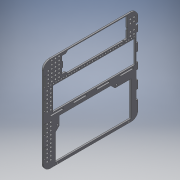
# Autodesk Inventor part: TrayPanelE
Saved by Autodesk Inventor 2017 (Build 210142000, 142)
## iProperties
Created: 2019-06-22
Part Number: TrayPanelE
Material: Generic
Document SubType Name: Modeling
Designer: DDeGo
Density: 1 g/cm^3
Appearance: Default
Author: DDeGo
Autodesk Inventor part; units mm, degrees
ref_plane "YZ Plane" through (0, 0, 0) normal (1, 0, 0) x (0, 1, 0)
ref_plane "XZ Plane" through (0, 0, 0) normal (0, 1, 0) x (-1, 0, 0)
ref_plane "XY Plane" through (0, 0, 0) normal (0, 0, 1) x (1, 0, 0)
sketch "Block1" plane through (0, 0, 0) normal (0, 0, 1) x (1, 0, 0)
  circle A0 centre (145, 9.5) radius 1.5
  circle A1 centre (31, 19.5) radius 1.5
  circle A2 centre (31, 83.5) radius 1.5
  circle A3 centre (169, 83.5) radius 1.5
  line L0 (27, 29.5) -> (27, 80.5)
  line L1 (27, 80.5) -> (173, 80.5)
  line L2 (173, 80.5) -> (173, 13.5)
  line L3 (173, 13.5) -> (142, 13.5)
  line L4 (142, 13.5) -> (134, 5.5)
  line L5 (134, 5.5) -> (34, 5.5)
  line L6 (34, 5.5) -> (34, 22.5)
  line L7 (34, 22.5) -> (27, 29.5)
  point P0 (93.25, 35.7812)
sketch "Sketch1" plane through (0, 0, 0) normal (1, 0, 0) x (0, 1, 0)
  line L0 (46.5, 144.8143) -> (46.5, 184.0143) construction
  line L1 (46.5, 184.0143) -> (162.5, 184.0143)
  line L2 (162.5, 184.0143) -> (162.5, 144.8143)
  line L3 (170, 185.4143) -> (13, 185.4143)
  arc A0 (13, 185.4143) -> (0, 172.4143) centre (13, 172.4143) ccw
  line L4 (0, 172.4143) -> (0, 15.4143)
  arc A1 (0, 15.4143) -> (13, 2.4143) centre (13, 15.4143) ccw
  line L5 (13, 2.4143) -> (170, 2.4143)
  arc A2 (170, 2.4143) -> (183, 15.4143) centre (170, 15.4143) ccw
  line L6 (183, 15.4143) -> (183, 172.4143)
  arc A3 (183, 172.4143) -> (170, 185.4143) centre (170, 172.4143) ccw
  line L7 (186.5, 14.4143) -> (186.5, 173.4143) projected
  arc A4 (186.5, 173.4143) -> (171, 188.9143) centre (171, 173.4143) ccw projected
  line L8 (171, 188.9143) -> (12, 188.9143) projected
  arc A5 (12, 188.9143) -> (-3.5, 173.4143) centre (12, 173.4143) ccw projected
  line L9 (-3.5, 173.4143) -> (-3.5, 14.4143) projected
  arc A6 (-3.5, 14.4143) -> (12, -1.0857) centre (12, 14.4143) ccw projected
  line L10 (12, -1.0857) -> (171, -1.0857) projected
  arc A7 (171, -1.0857) -> (186.5, 14.4143) centre (171, 14.4143) ccw projected
  arc A8 (46.5, 184.0143) -> (46.1505, 183.8718) centre (46.5, 183.5143) ccw
  line L11 (46.1505, 183.8718) -> (42.3495, 180.1567)
  arc A9 (42, 180.0143) -> (42.3495, 180.1567) centre (42, 180.5143) ccw
  line L12 (42, 180.0143) -> (35.5, 180.0143)
  arc A10 (35.5, 180.0143) -> (34.5, 179.0143) centre (35.5, 179.0143) ccw
  line L13 (34.5, 179.0143) -> (34.5, 170.4143)
  arc A11 (34.5, 170.4143) -> (35.5, 169.4143) centre (35.5, 170.4143) ccw
  line L14 (35.5, 169.4143) -> (37, 169.4143)
  line L15 (37, 159.4143) -> (35.5, 159.4143)
  arc A12 (35.5, 159.4143) -> (34.5, 158.4143) centre (35.5, 158.4143) ccw
  line L16 (34.5, 158.4143) -> (34.5, 149.8143)
  arc A13 (34.5, 149.8143) -> (35.5, 148.8143) centre (35.5, 149.8143) ccw
  line L17 (35.5, 148.8143) -> (42, 148.8143)
  arc A14 (42.3495, 148.6718) -> (42, 148.8143) centre (42, 148.3143) ccw
  line L18 (42.3495, 148.6718) -> (46.1505, 144.9567)
  arc A15 (46.1505, 144.9567) -> (46.5, 144.8143) centre (46.5, 145.3143) ccw
  line L19 (37, 169.4143) -> (37, 159.4143)
  line L20 (177.5, 93.9143) -> (18.5, 93.9143)
  line L21 (18.5, 93.9143) -> (18.5, 138.6143)
  line L22 (18.5, 138.6143) -> (177.5, 138.6143)
  line L23 (177.5, 138.6143) -> (177.5, 93.9143)
  line L24 (156.5, 144.8143) -> (156.5, 141.3143)
  line L25 (156.5, 141.3143) -> (155, 141.3143)
  line L26 (155, 141.3143) -> (155, 144.8143)
  line L27 (162.5, 144.8143) -> (156.5, 144.8143)
  line L28 (155, 144.8143) -> (46.5, 144.8143)
  line L29 (37, 164.4143) -> (41, 164.4143) construction
  circle A16 centre (41, 164.4143) radius 1.5 construction
  line L30 (37.5, 154.4143) -> (44.5, 154.4143) construction
  line L31 (44.5, 154.4143) -> (44.5, 174.4143) construction
  line L32 (44.5, 174.4143) -> (37.5, 174.4143) construction
  line L33 (37.5, 174.4143) -> (37.5, 154.4143) construction
  line L34 (37.5, 154.4143) -> (44.5, 174.4143) construction
  line L35 (44.5, 154.4143) -> (37.5, 174.4143) construction
  line L36 (169.5, 77.9143) -> (138.5, 77.9143)
  circle A17 centre (141.5, 81.9143) radius 2.25
  line L37 (138.5, 77.9143) -> (130.5, 85.9143)
  line L38 (130.5, 85.9143) -> (30.5, 85.9143)
  circle A18 centre (27.5, 71.9143) radius 2.25
  line L39 (30.5, 85.9143) -> (30.5, 68.9143)
  line L40 (30.5, 68.9143) -> (23.5, 61.9143)
  line L41 (23.5, 61.9143) -> (23.5, 10.9143)
  circle A19 centre (27.5, 7.9143) radius 2.25
  line L42 (23.5, 10.9143) -> (169.5, 10.9143)
  circle A20 centre (165.5, 7.9143) radius 2.25
  line L43 (169.5, 10.9143) -> (169.5, 77.9143)
  point P0 (46.5, 164.4143)
  point P1 (-6.081, 1.5)
  dimension "d3" = 183
  dimension "d5" = 13
  dimension "d10" = 10.6
  dimension "d11" = 10.6
  dimension "d12" = 10
  dimension "d17" = 4
  dimension "d18" = 0.5
  dimension "d19" = 1
  dimension "d55" = 183
  dimension "d57" = 3.5
  dimension "d63" = 18.5
  dimension "d64" = 91.5
  dimension "d65" = 44.7
  dimension "d66" = 159
  dimension "d67" = 3.5
  dimension "d85" = 20.5
  dimension "d86" = 1.4
  dimension "d87" = 116
  dimension "d88" = 4
  dimension "d89" = 3.5
  dimension "d90" = 6
  dimension "d91" = 1.5
  dimension "d92" = 12
  dimension "d93" = 2.5
  dimension "d94" = 4.5
  dimension "d95" = 4.5
  dimension "d96" = 3
  dimension "d97" = 7
  dimension "d98" = 4
  dimension "d99" = 20
  dimension "d103" = 122
  constraints: 80 end point, 25 tangent, 24 point on circle, 17 centre point, 11 horizontal, 9 equal radius, 8 perpendicular, 6 vertical, 4 midpoint, 4 parallel, 1 coincident, 1 collinear, 18 other
  measures "d3" distance between parallel lines of L3 L5
  measures "d5" radius of A0
  measures "d10" distance between parallel lines of L12 L14
  measures "d11" distance between parallel lines of L17 L15
  measures "d12" distance between parallel lines of L14 L15
  measures "d17" distance between parallel lines of L1 L12
  measures "d18" radius of A14
  measures "d19" radius of A13
  measures "d55" distance between parallel lines of L6 L4
  measures "d57" distance between parallel lines of L9 L4
  measures "d63" distance between parallel lines of L4 L21
  measures "d64" distance between parallel lines of L5 L20
  measures "d65" distance between parallel lines of L22 L20
  measures "d66" distance between parallel lines of L23 L21
  measures "d67" distance between parallel lines of L10 L5
  measures "d85" distance between parallel lines of L6 L2
  measures "d86" distance between parallel lines of L3 L1
  measures "d87" distance between parallel lines of L2 L0
  measures "d88" distance between parallel lines of L17 L28
  measures "d89" distance between parallel lines of L28 L25
  measures "d90" distance between parallel lines of L24 L2
  measures "d91" distance between parallel lines of L26 L24
  measures "d92" distance between parallel lines of L0 L13
  measures "d93" distance between parallel lines of L13 L19
  measures "d94" distance from line of L0 L12.start
  measures "d95" distance from line of L0 L17.end
  measures "d96" diameter of A16
  measures "d97" distance of L30.start L30.end
  measures "d98" distance of L29.start L29.end
  measures "d99" distance of L30.end L31.end
  measures "d103" distance between parallel lines of L13 L24
extrude "Extrusion1" add sketch "Sketch1" along normal blind 2.75 contours A3 L6 A2 L5 A1 L4 A0 L3
sketch "Sketch2" plane through (2.75, 0, 0) normal (1, 0, 0) x (0, 0, -1)
  line L0 (-91.375, 13.5) -> (-88.625, 13.5)
  line L1 (-88.625, 13.5) -> (-88.625, 38.5)
  line L2 (-88.625, 38.5) -> (-91.375, 38.5)
  line L3 (-91.375, 38.5) -> (-91.375, 13.5)
  line L4 (-91.375, 58.5) -> (-88.625, 58.5)
  line L5 (-88.625, 58.5) -> (-88.625, 83.5)
  line L6 (-88.625, 83.5) -> (-91.375, 83.5)
  line L7 (-91.375, 83.5) -> (-91.375, 58.5)
  line L8 (-91.375, 103.5) -> (-88.625, 103.5)
  line L9 (-88.625, 103.5) -> (-88.625, 128.5)
  line L10 (-88.625, 128.5) -> (-91.375, 128.5)
  line L11 (-91.375, 128.5) -> (-91.375, 103.5)
  line L12 (-91.375, 148.5) -> (-88.625, 148.5)
  line L13 (-88.625, 148.5) -> (-88.625, 173.5)
  line L14 (-88.625, 173.5) -> (-91.375, 173.5)
  line L15 (-91.375, 173.5) -> (-91.375, 148.5)
  line L16 (-162, 1.625) -> (-142, 1.625)
  line L17 (-142, 1.625) -> (-142, 4.375)
  line L18 (-142, 4.375) -> (-162, 4.375)
  line L19 (-162, 4.375) -> (-162, 1.625)
  line L20 (-122, 1.625) -> (-102, 1.625)
  line L21 (-102, 1.625) -> (-102, 4.375)
  line L22 (-102, 4.375) -> (-122, 4.375)
  line L23 (-122, 4.375) -> (-122, 1.625)
  line L24 (-82, 1.625) -> (-62, 1.625)
  line L25 (-62, 1.625) -> (-62, 4.375)
  line L26 (-62, 4.375) -> (-82, 4.375)
  line L27 (-82, 4.375) -> (-82, 1.625)
  line L28 (-42, 1.625) -> (-22, 1.625)
  line L29 (-22, 1.625) -> (-22, 4.375)
  line L30 (-22, 4.375) -> (-42, 4.375)
  line L31 (-42, 4.375) -> (-42, 1.625)
  line L32 (-15.4143, 183) -> (-172.4143, 183) projected
  line L33 (-172.4143, 0) -> (-15.4143, 0) projected
  line L34 (-185.4143, 170) -> (-185.4143, 13) projected
  point P0 (0, 0)
  point P1 (-90, 128.5)
  point P2 (-142, 3)
  dimension "d22" = 25
  dimension "d23" = 2.75
  dimension "d24" = 9.5
  dimension "d29" = 90
  dimension "d30" = 2.75
  dimension "d31" = 3
  dimension "d32" = 22
  dimension "d36" = 20
  dimension "d37" = 23.4143
  dimension "d38" = 9.125
  dimension "d41" = 45
  dimension "d42" = 45
  dimension "d43" = 45
  dimension "d44" = 40
  dimension "d45" = 40
  dimension "d46" = 40
  constraints: 64 end point, 16 parallel, 12 point on line, 8 horizontal, 8 perpendicular, 6 collinear, 2 midpoint
  measures "d22" distance of L2.end L0.start
  measures "d23" distance of L13.end L14.end
  measures "d24" distance between parallel lines of L14 L32
  measures "d29" horizontal distance of point (0, 0) point (-90, 128.5)
  measures "d30" distance of L18.end L16.start
  measures "d31" vertical distance of point (0, 0) point (-142, 3)
  measures "d32" horizontal distance of L29.end point (0, 0)
  measures "d36" distance of L17.end L18.end
  measures "d37" distance between parallel lines of L34 L19
  measures "d38" distance between parallel lines of L22 L0
  measures "d41" distance of L10.end L14.end
  measures "d42" distance of L6.end L10.end
  measures "d43" distance of L2.end L6.end
  measures "d44" distance of L25.end L29.end
  measures "d45" distance of L21.end L25.end
  measures "d46" distance of L17.end L21.end
extrude "Extrusion2" cut sketch "Sketch2" against normal blind 10
sketch "Sketch3" plane through (2.75, 0, 0) normal (1, 0, 0) x (0, 0, -1)
  line L0 (-15.4143, 183) -> (-172.4143, 183) projected
  line L1 (-114, 183) -> (-96, 183)
  line L2 (-96, 183) -> (-96, 179.5)
  line L3 (-96, 179.5) -> (-114, 179.5)
  line L4 (-114, 179.5) -> (-114, 183)
  line L5 (-129, 183) -> (-147, 183)
  line L6 (-147, 183) -> (-147, 179.5)
  line L7 (-147, 179.5) -> (-129, 179.5)
  line L8 (-129, 179.5) -> (-129, 183)
  line L9 (-84, 183) -> (-66, 183)
  line L10 (-66, 183) -> (-66, 179.5)
  line L11 (-66, 179.5) -> (-84, 179.5)
  line L12 (-84, 179.5) -> (-84, 183)
  line L13 (-51, 183) -> (-33, 183)
  line L14 (-33, 183) -> (-33, 179.5)
  line L15 (-33, 179.5) -> (-51, 179.5)
  line L16 (-51, 179.5) -> (-51, 183)
  line L17 (-91.375, 173.5) -> (-88.625, 173.5) projected
  line L18 (-90, 173.5) -> (-90, 183) construction
  point P0 (0, 0)
  dimension "d47" = 18
  dimension "d48" = 3.5
  dimension "d49" = 6
  dimension "d50" = 15
  dimension "d51" = 6
  dimension "d52" = 15
  constraints: 34 end point, 8 parallel, 8 point on line, 5 perpendicular, 4 horizontal, 3 collinear, 1 midpoint
  measures "d47" distance of L14.end L15.end
  measures "d48" distance of L5.end L6.end
  measures "d49" distance between parallel lines of L12 L18
  measures "d50" distance between parallel lines of L10 L16
  measures "d51" distance between parallel lines of L2 L18
  measures "d52" distance between parallel lines of L8 L4
extrude "Extrusion3" cut sketch "Sketch3" against normal blind 10
sketch "Sketch5" plane through (0, 0, 0) normal (-1, 0, 0) x (0, 0, 1)
  line L0 (172.4143, 183) -> (147, 183) projected
  line L1 (163.0643, 183) -> (158.7643, 183)
  line L2 (158.7643, 183) -> (158.7643, 178.5)
  line L3 (158.7643, 178.5) -> (163.0643, 178.5)
  line L4 (163.0643, 178.5) -> (163.0643, 183)
  line L5 (144.8143, 156.5) -> (144.8143, 162.5) projected
  line L6 (144.8143, 162.5) -> (184.0143, 162.5) projected
  line L7 (163.0643, 162.5) -> (158.7643, 162.5)
  line L8 (158.7643, 162.5) -> (158.7643, 163.5)
  line L9 (158.7643, 163.5) -> (163.0643, 163.5)
  line L10 (163.0643, 163.5) -> (163.0643, 162.5)
  point P0 (0, 0)
  point P1 (160.9143, 178.5)
  point P2 (144.5143, 47.5)
  point P3 (185.4143, 158)
  dimension "d70" = 16.1
  dimension "d71" = 4.3
  dimension "d72" = 4.5
  dimension "d75" = 1
  constraints: 16 end point, 4 parallel, 2 collinear, 2 horizontal, 2 perpendicular, 1 midpoint, 1 point on line, 3 other
  measures "d71" distance between parallel lines of L4 L2
  measures "d72" distance between parallel lines of L0 L3
extrude "Extrusion5" cut sketch "Sketch5" against normal blind 10
sketch "Sketch6" plane through (0, 0, 0) normal (-1, 0, 0) x (0, 0, 1)
  line L0 (178.4143, 176) -> (9.4143, 176) construction
  line L1 (9.4143, 176) -> (9.4143, 7) construction
  line L2 (9.4143, 7) -> (178.4143, 7) construction
  line L3 (178.4143, 7) -> (178.4143, 176) construction
  line L4 (2.4143, 170) -> (2.4143, 13) construction
  line L5 (33, 183) -> (15.4143, 183) construction
  line L6 (185.4143, 13) -> (185.4143, 170) construction
  line L7 (15.4143, 0) -> (172.4143, 0) construction
  circle A0 centre (178.4143, 176) radius 2.05
  circle A1 centre (178.4143, 7) radius 2.05
  circle A2 centre (9.4143, 7) radius 2.05
  circle A3 centre (9.4143, 176) radius 2.05
  point P0 (0, 0)
  dimension "d76" = 7
  dimension "d77" = 7
  dimension "d78" = 7
  dimension "d79" = 7
  dimension "d80" = 4.1
  constraints: 8 end point, 4 centre point, 4 coincident, 3 equal radius, 2 parallel, 1 horizontal, 1 perpendicular
  measures "d76" distance between parallel lines of L4 L1
  measures "d77" distance between parallel lines of L5 L0
  measures "d78" distance between parallel lines of L6 L3
  measures "d79" distance between parallel lines of L7 L2
  measures "d80" diameter of A0
extrude "Extrusion6" [suppressed]
sketch "Sketch7" plane through (0, 0, 0) normal (-1, 0, 0) x (0, 0, 1)
  circle A0 centre (174.9143, 175.5) radius 2
  circle A1 centre (174.9143, 168.5) radius 2
  circle A2 centre (167.9143, 168.5) radius 2
  circle A3 centre (167.9143, 175.5) radius 2
  circle A4 centre (153.9143, 175.5) radius 2
  circle A5 centre (153.9143, 168.5) radius 2
  circle A6 centre (146.9143, 175.5) radius 2
  circle A7 centre (146.9143, 168.5) radius 2
  circle A8 centre (141.7643, 175.5) radius 1.5
  circle A9 centre (141.7643, 170.4697) radius 1.5
  circle A10 centre (141.7643, 165.4394) radius 1.5
  circle A11 centre (141.7643, 160.4091) radius 1.5
  circle A12 centre (141.7643, 150.3485) radius 1.5
  circle A13 centre (141.7643, 145.3182) radius 1.5
  circle A14 centre (141.7643, 140.2879) radius 1.5
  circle A15 centre (141.7643, 135.2576) radius 1.5
  circle A16 centre (141.7643, 130.2273) radius 1.5
  circle A17 centre (141.7643, 125.197) radius 1.5
  circle A18 centre (141.7643, 120.1667) radius 1.5
  circle A19 centre (141.7643, 115.1364) radius 1.5
  circle A20 centre (141.7643, 110.1061) radius 1.5
  circle A21 centre (141.7643, 105.0758) radius 1.5
  circle A22 centre (141.7643, 100.0455) radius 1.5
  circle A23 centre (141.7643, 95.0152) radius 1.5
  circle A24 centre (141.7643, 89.9848) radius 1.5
  circle A25 centre (141.7643, 84.9545) radius 1.5
  circle A26 centre (141.7643, 79.9242) radius 1.5
  circle A27 centre (141.7643, 74.8939) radius 1.5
  line L0 (163.0643, 183) -> (163.0643, 178.5) projected
  line L1 (163.0643, 178.5) -> (158.7643, 178.5) projected
  line L2 (158.7643, 178.5) -> (158.7643, 183) projected
  line L3 (158.7643, 183) -> (147, 183) projected
  line L4 (147, 183) -> (147, 179.5) projected
  line L5 (147, 179.5) -> (129, 179.5) projected
  line L6 (129, 179.5) -> (129, 183) projected
  line L7 (129, 183) -> (114, 183) projected
  line L8 (114, 183) -> (114, 179.5) projected
  line L9 (114, 179.5) -> (96, 179.5) projected
  line L10 (96, 179.5) -> (96, 183) projected
  line L11 (96, 183) -> (84, 183) projected
  line L12 (84, 183) -> (84, 179.5) projected
  line L13 (84, 179.5) -> (66, 179.5) projected
  line L14 (66, 179.5) -> (66, 183) projected
  line L15 (66, 183) -> (51, 183) projected
  line L16 (51, 183) -> (51, 179.5) projected
  line L17 (51, 179.5) -> (33, 179.5) projected
  line L18 (33, 179.5) -> (33, 183) projected
  line L19 (33, 183) -> (15.4143, 183) projected
  arc A28 (15.4143, 183) -> (2.4143, 170) centre (15.4143, 170) ccw projected
  line L20 (2.4143, 170) -> (2.4143, 13) projected
  arc A29 (2.4143, 13) -> (15.4143, 0) centre (15.4143, 13) ccw projected
  line L21 (15.4143, 0) -> (172.4143, 0) projected
  arc A30 (172.4143, 0) -> (185.4143, 13) centre (172.4143, 13) ccw projected
  line L22 (185.4143, 13) -> (185.4143, 170) projected
  arc A31 (185.4143, 170) -> (172.4143, 183) centre (172.4143, 170) ccw projected
  line L23 (172.4143, 183) -> (163.0643, 183) projected
  line L24 (158.7643, 162.5) -> (158.7643, 163.5) projected
  line L25 (158.7643, 163.5) -> (163.0643, 163.5) projected
  line L26 (163.0643, 163.5) -> (163.0643, 162.5) projected
  line L27 (163.0643, 162.5) -> (184.0143, 162.5) projected
  line L28 (184.0143, 162.5) -> (184.0143, 46.5) projected
  arc A32 (183.8718, 46.1505) -> (184.0143, 46.5) centre (183.5143, 46.5) ccw projected
  line L29 (183.8718, 46.1505) -> (180.1567, 42.3495) projected
  arc A33 (180.1567, 42.3495) -> (180.0143, 42) centre (180.5143, 42) ccw projected
  line L30 (180.0143, 42) -> (180.0143, 35.5) projected
  arc A34 (179.0143, 34.5) -> (180.0143, 35.5) centre (179.0143, 35.5) ccw projected
  line L31 (179.0143, 34.5) -> (170.4143, 34.5) projected
  arc A35 (169.4143, 35.5) -> (170.4143, 34.5) centre (170.4143, 35.5) ccw projected
  line L32 (169.4143, 35.5) -> (169.4143, 37) projected
  line L33 (169.4143, 37) -> (159.4143, 37) projected
  line L34 (159.4143, 37) -> (159.4143, 35.5) projected
  arc A36 (158.4143, 34.5) -> (159.4143, 35.5) centre (158.4143, 35.5) ccw projected
  line L35 (158.4143, 34.5) -> (149.8143, 34.5) projected
  arc A37 (148.8143, 35.5) -> (149.8143, 34.5) centre (149.8143, 35.5) ccw projected
  line L36 (148.8143, 35.5) -> (148.8143, 42) projected
  arc A38 (148.8143, 42) -> (148.6718, 42.3495) centre (148.3143, 42) ccw projected
  line L37 (148.6718, 42.3495) -> (144.9567, 46.1505) projected
  arc A39 (144.8143, 46.5) -> (144.9567, 46.1505) centre (145.3143, 46.5) ccw projected
  line L38 (144.8143, 46.5) -> (144.8143, 155) projected
  line L39 (144.8143, 155) -> (141.3143, 155) projected
  line L40 (141.3143, 155) -> (141.3143, 156.5) projected
  line L41 (141.3143, 156.5) -> (144.8143, 156.5) projected
  line L42 (144.8143, 156.5) -> (144.8143, 162.5) projected
  line L43 (144.8143, 162.5) -> (158.7643, 162.5) projected
  line L44 (138.6143, 18.5) -> (93.9143, 18.5) projected
  line L45 (93.9143, 18.5) -> (93.9143, 177.5) projected
  line L46 (93.9143, 177.5) -> (138.6143, 177.5) projected
  line L47 (138.6143, 177.5) -> (138.6143, 18.5) projected
  line L48 (22, 1.625) -> (22, 4.375) projected
  line L49 (22, 4.375) -> (42, 4.375) projected
  line L50 (42, 4.375) -> (42, 1.625) projected
  line L51 (42, 1.625) -> (22, 1.625) projected
  line L52 (102, 1.625) -> (102, 4.375) projected
  line L53 (102, 4.375) -> (122, 4.375) projected
  line L54 (122, 4.375) -> (122, 1.625) projected
  line L55 (122, 1.625) -> (102, 1.625) projected
  line L56 (88.625, 148.5) -> (88.625, 173.5) projected
  line L57 (88.625, 173.5) -> (91.375, 173.5) projected
  line L58 (91.375, 173.5) -> (91.375, 148.5) projected
  line L59 (91.375, 148.5) -> (88.625, 148.5) projected
  line L60 (88.625, 58.5) -> (88.625, 83.5) projected
  line L61 (88.625, 83.5) -> (91.375, 83.5) projected
  line L62 (91.375, 83.5) -> (91.375, 58.5) projected
  line L63 (91.375, 58.5) -> (88.625, 58.5) projected
  line L64 (88.625, 13.5) -> (88.625, 38.5) projected
  line L65 (88.625, 38.5) -> (91.375, 38.5) projected
  line L66 (91.375, 38.5) -> (91.375, 13.5) projected
  line L67 (91.375, 13.5) -> (88.625, 13.5) projected
  line L68 (88.625, 103.5) -> (88.625, 128.5) projected
  line L69 (88.625, 128.5) -> (91.375, 128.5) projected
  line L70 (91.375, 128.5) -> (91.375, 103.5) projected
  line L71 (91.375, 103.5) -> (88.625, 103.5) projected
  line L72 (142, 1.625) -> (142, 4.375) projected
  line L73 (142, 4.375) -> (162, 4.375) projected
  line L74 (162, 4.375) -> (162, 1.625) projected
  line L75 (162, 1.625) -> (142, 1.625) projected
  line L76 (62, 1.625) -> (62, 4.375) projected
  line L77 (62, 4.375) -> (82, 4.375) projected
  line L78 (82, 4.375) -> (82, 1.625) projected
  line L79 (82, 1.625) -> (62, 1.625) projected
  circle A40 centre (141.7643, 64.8333) radius 1.5
  circle A41 centre (141.7643, 69.8636) radius 1.5
  circle A42 centre (141.7643, 59.803) radius 1.5
  circle A43 centre (141.7643, 54.7727) radius 1.5
  circle A44 centre (141.7643, 49.7424) radius 1.5
  circle A45 centre (141.7643, 44.7121) radius 1.5
  circle A46 centre (141.7643, 39.6818) radius 1.5
  circle A47 centre (141.7643, 34.6515) radius 1.5
  circle A48 centre (146.9143, 30.5) radius 2
  circle A49 centre (153.9143, 30.5) radius 2
  circle A50 centre (167.9143, 30.5) radius 2
  circle A51 centre (160.9143, 30.5) radius 2
  circle A52 centre (160.9143, 23.5) radius 2
  circle A53 centre (167.9143, 23.5) radius 2
  circle A54 centre (167.9143, 16.5) radius 2
  circle A55 centre (167.9143, 9.5) radius 2
  circle A56 centre (160.9143, 9.5) radius 2
  circle A57 centre (160.9143, 16.5) radius 2
  circle A58 centre (153.9143, 16.5) radius 2
  circle A59 centre (153.9143, 9.5) radius 2
  circle A60 centre (146.9143, 9.5) radius 2
  circle A61 centre (146.9143, 16.5) radius 2
  circle A62 centre (146.9143, 23.5) radius 2
  circle A63 centre (153.9143, 23.5) radius 2
  circle A64 centre (141.7643, 29.6212) radius 1.5
  circle A65 centre (141.7643, 24.5909) radius 1.5
  circle A66 centre (141.7643, 19.5606) radius 1.5
  circle A67 centre (141.7643, 14.5303) radius 1.5
  circle A68 centre (141.7643, 9.5) radius 1.5
  circle A69 centre (181.9143, 30.5) radius 2
  circle A70 centre (174.9143, 30.5) radius 2
  circle A71 centre (174.9143, 23.5) radius 2
  circle A72 centre (181.9143, 23.5) radius 2
  circle A73 centre (181.9143, 16.5) radius 2
  circle A74 centre (174.9143, 16.5) radius 2
  circle A75 centre (135.4643, 14.5) radius 2
  circle A76 centre (135.4643, 7.5) radius 2
  circle A77 centre (128.4643, 7.5) radius 2
  circle A78 centre (128.4643, 14.5) radius 2
  circle A79 centre (121.4643, 7.5) radius 2
  circle A80 centre (121.4643, 14.5) radius 2
  circle A81 centre (114.4643, 14.5) radius 2
  circle A82 centre (114.4643, 7.5) radius 2
  circle A83 centre (107.4643, 7.5) radius 2
  circle A84 centre (107.4643, 14.5) radius 2
  circle A85 centre (100.4643, 14.5) radius 2
  circle A86 centre (100.4643, 7.5) radius 2
  circle A87 centre (16.4643, 7.5) radius 2
  circle A88 centre (16.4643, 14.5) radius 2
  circle A89 centre (23.4643, 14.5) radius 2
  circle A90 centre (23.4643, 7.5) radius 2
  circle A91 centre (30.4643, 14.5) radius 2
  circle A92 centre (30.4643, 7.5) radius 2
  circle A93 centre (37.4643, 7.5) radius 2
  circle A94 centre (37.4643, 14.5) radius 2
  circle A95 centre (44.4643, 14.5) radius 2
  circle A96 centre (44.4643, 7.5) radius 2
  circle A97 centre (51.4643, 14.5) radius 2
  circle A98 centre (51.4643, 7.5) radius 2
  circle A99 centre (58.4643, 14.5) radius 2
  circle A100 centre (58.4643, 7.5) radius 2
  circle A101 centre (65.4643, 14.5) radius 2
  circle A102 centre (65.4643, 7.5) radius 2
  circle A103 centre (72.4643, 14.5) radius 2
  circle A104 centre (72.4643, 7.5) radius 2
  circle A105 centre (79.4643, 14.5) radius 2
  circle A106 centre (79.4643, 7.5) radius 2
  point P0 (0, 0)
  constraints: 95 centre point, 190 other
extrude "Extrusion7" cut sketch "Sketch7" against normal blind 10 contours A0 | A1 | A2 | A3 | A4 | A5 | A6 | A7 | A8 | A9 | A10 | A11 | A12 | A13 | A14 | A15 | A16 | A17 | A18 | A19 | A20 | A21 | A22 | A23 | A24 | A25 | A26 | A27 | A40 | A41 | A42 | A43 | A44 | A45 | A46 | A47 | A48 | A49 | A50 | A51 | A52 | A53 | A54 | A55 | A56 | A57 | A58 | A59 | A60 | A61 | A62 | A63 | A64 | A65 | A66 | A67 | A68 | A69 | A70 | A71 | A72 | A73 | A74 | A75 | A76 | A77 | A78 | A79 | A80 | A81 | A82 | A83 | A84 | A85 | A86 | A87 | A88 | A89 | A90 | A91 | A92 | A93 | A94 | A95 | A96 | A97 | A98 | A99 | A100 | A101 | A102 | A103 | A104 | A105 | A106
body "Solid1"
